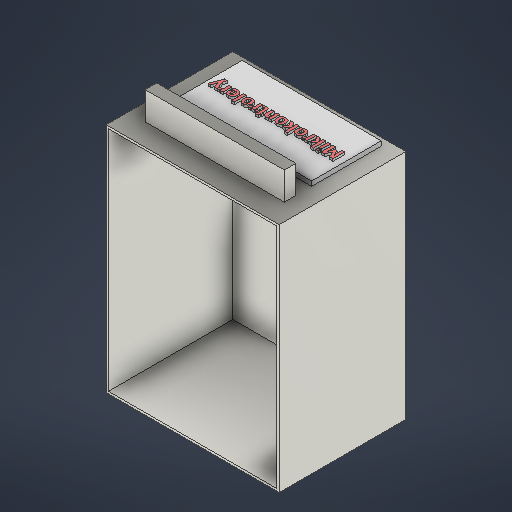
# Autodesk Inventor part: shelf
Saved by Autodesk Inventor 2027 (Build 310192060, 192F)
## iProperties
Created: 2026-06-08
Part Number: shelf
Material: Ogólny
Document SubType Name: Modeling
Designer: User
Density: 1 g/cm^3
Appearance: Domyślna
Author: User
Autodesk Inventor part; units mm, degrees
ref_plane "YZ Plane" through (0, 0, 0) normal (1, 0, 0) x (0, 1, 0)
ref_plane "XZ Plane" through (0, 0, 0) normal (0, 1, 0) x (-1, 0, 0)
ref_plane "XY Plane" through (0, 0, 0) normal (0, 0, 1) x (1, 0, 0)
sketch "Szkic1" plane through (0, 0, 0) normal (0, 1, 0) x (-1, 0, 0)
  line L0 (-37.3, -27.3) -> (37.3, -27.3)
  line L1 (37.3, -27.3) -> (37.3, 27.3)
  line L2 (37.3, 27.3) -> (-37.3, 27.3)
  line L3 (-37.3, 27.3) -> (-37.3, -27.3)
  line L4 (-37.3, -27.3) -> (37.3, 27.3) construction
  line L5 (37.3, -27.3) -> (-37.3, 27.3) construction
  point P0 (0, 0)
  dimension "d0" = 74.6
  dimension "d1" = 54.6
  constraints: 12 end point, 2 midpoint, 2 parallel, 1 horizontal, 1 perpendicular
  measures "d0" distance of L2.end L1.end
  measures "d1" distance of L1.end L0.end
extrude "Wyciągnięcie proste1" add sketch "Szkic1" along normal blind 100
shell "Skorupa1" thickness 1 removed faces 1 at (-12.4333, 33.3333, 27.3)
sketch "Szkic2" plane through (0, 100, 0) normal (0, 1, 0) x (1, 0, 0)
  line L0 (-37.3, -27.3) -> (37.3, -27.3) projected
  line L1 (0, -27.3) -> (0, -15.3)
  line L2 (30, -17.8) -> (-30, -17.8)
  line L3 (-30, -17.8) -> (-30, -12.8)
  line L4 (-30, -12.8) -> (30, -12.8)
  line L5 (30, -12.8) -> (30, -17.8)
  line L6 (30, -17.8) -> (-30, -12.8) construction
  line L7 (-30, -17.8) -> (30, -12.8) construction
  point P0 (0, 0)
  dimension "d5" = 12
  dimension "d6" = 60
  dimension "d7" = 5
  constraints: 14 end point, 3 midpoint, 2 parallel, 1 horizontal, 1 perpendicular, 1 vertical
  measures "d5" distance of L1.start L1.end
  measures "d6" distance of L2.start L2.end
  measures "d7" distance of L2.end L3.end
extrude "Wyciągnięcie proste2" add sketch "Szkic2" along normal blind 12
sketch "Szkic3" plane through (0, 100, 0) normal (0, 1, 0) x (1, 0, 0)
  line L0 (0, 0) -> (0, 9)
  line L1 (30, 24) -> (-30, 24)
  line L2 (-30, 24) -> (-30, -6)
  line L3 (-30, -6) -> (30, -6)
  line L4 (30, -6) -> (30, 24)
  line L5 (30, 24) -> (-30, -6) construction
  line L6 (-30, 24) -> (30, -6) construction
  dimension "d10" = 9
  dimension "d11" = 60
  dimension "d12" = 30
  constraints: 14 end point, 2 midpoint, 2 parallel, 1 horizontal, 1 perpendicular, 1 vertical
  measures "d10" distance of L0.start L0.end
  measures "d11" distance of L3.end L2.end
  measures "d12" distance of L2.end L1.end
extrude "Wyciągnięcie proste3" add sketch "Szkic3" along normal blind 2
sketch "Szkic4" plane through (0, 102, 0) normal (0, 1, 0) x (1, 0, 0)
  line L0 (30, -6) -> (-30, -6) construction
  line L1 (-30, -6) -> (-30, 24) construction
  line L2 (-30, 24) -> (30, 24) construction
  line L3 (30, 24) -> (30, -6) construction
  line L4 (-30, -6) -> (30, -6) projected
  line L5 (-30, 24) -> (-30, -6) projected
  line L6 (30, -6) -> (-30, -6)
  line L7 (-30, -6) -> (-30, 24)
  line L8 (-30, 24) -> (30, 24)
  line L9 (30, 24) -> (30, -6)
  line L10 (22.1617, 10.9226) -> (23.4096, 10.9226)
  line L11 (23.4096, 10.9226) -> (23.4096, 7.6082)
  line L12 (23.4096, 7.6082) -> (24.3173, 9.7476)
  line L13 (24.3173, 9.7476) -> (25.1763, 9.7476)
  line L14 (25.1763, 9.7476) -> (26.0839, 7.6082)
  line L15 (26.0839, 7.6082) -> (26.0839, 10.9226)
  line L16 (26.0839, 10.9226) -> (27.267, 10.9226)
  line L17 (27.267, 10.9226) -> (27.267, 5.9226)
  line L18 (27.267, 5.9226) -> (25.8205, 5.9226)
  line L19 (25.8205, 5.9226) -> (24.7103, 8.3902)
  line L20 (24.7103, 8.3902) -> (23.6082, 5.9226)
  line L21 (23.6082, 5.9226) -> (22.1617, 5.9226)
  line L22 (22.1617, 5.9226) -> (22.1617, 10.9226)
  line L23 (20.0182, 10.9226) -> (21.1933, 10.9226)
  line L24 (21.1933, 10.9226) -> (21.1933, 7.1503)
  line L25 (21.1933, 7.1503) -> (20.0182, 7.1503)
  line L26 (20.0182, 7.1503) -> (20.0182, 10.9226)
  line L27 (19.9818, 6.6114) -> (21.2257, 6.6114)
  line L28 (21.2257, 6.6114) -> (21.2257, 5.6957)
  line L29 (21.2257, 5.6957) -> (19.9818, 5.6957)
  line L30 (19.9818, 5.6957) -> (19.9818, 6.6114)
  line L31 (15.3424, 10.9226) -> (16.7403, 10.9226)
  line L32 (16.7403, 10.9226) -> (17.7613, 9.2857)
  line L33 (17.7613, 9.2857) -> (17.9437, 9.5288)
  line L34 (17.9437, 9.5288) -> (17.9437, 10.9226)
  line L35 (17.9437, 10.9226) -> (19.1187, 10.9226)
  line L36 (19.1187, 10.9226) -> (19.1187, 5.6998)
  line L37 (19.1187, 5.6998) -> (17.9437, 5.6998)
  line L38 (17.9437, 5.6998) -> (17.9437, 8.6252)
  line L39 (17.9437, 8.6252) -> (16.8294, 7.1503)
  line L40 (16.8294, 7.1503) -> (15.4396, 7.1503)
  line L41 (15.4396, 7.1503) -> (16.7605, 8.7751)
  line L42 (16.7605, 8.7751) -> (15.3424, 10.9226)
  line L43 (12.4412, 8.2646) -> (12.5385, 8.2646)
  spline S0 degree 2 poles (12.5385, 8.2646) (12.6074, 8.2403) (12.8626, 8.216) (13.0166, 8.216) knots 0 0 0 1 2 2 2
  spline S1 degree 2 poles (13.0166, 8.216) (13.1989, 8.216) (13.6082, 8.3254) (13.7986, 8.3983) knots 0 0 0 1 2 2 2
  line L44 (13.7986, 8.3983) -> (13.7986, 10.9226)
  line L45 (13.7986, 10.9226) -> (14.9737, 10.9226)
  line L46 (14.9737, 10.9226) -> (14.9737, 7.1503)
  line L47 (14.9737, 7.1503) -> (13.7986, 7.1503)
  line L48 (13.7986, 7.1503) -> (13.7986, 7.6933)
  spline S2 degree 2 poles (13.7986, 7.6933) (13.7176, 7.6203) (13.434, 7.3934) (13.3165, 7.3246) knots 0 0 0 1 2 2 2
  spline S3 degree 2 poles (13.3165, 7.3246) (13.1868, 7.2476) (12.8464, 7.1382) (12.6965, 7.1382) knots 0 0 0 1 2 2 2
  spline S4 degree 2 poles (12.6965, 7.1382) (12.6398, 7.1382) (12.498, 7.1463) (12.4412, 7.1503) knots 0 0 0 1 2 2 2
  line L49 (12.4412, 7.1503) -> (12.4412, 8.2646)
  spline S5 degree 2 poles (8.3732, 9.0385) (8.3732, 9.9704) (9.3902, 11.0401) (10.3181, 11.0401) knots 0 0 0 1 2 2 2
  spline S6 degree 2 poles (10.3181, 11.0401) (11.2419, 11.0401) (12.267, 9.9704) (12.267, 9.0385) knots 0 0 0 1 2 2 2
  spline S7 degree 2 poles (12.267, 9.0385) (12.267, 8.0985) (11.2419, 7.0328) (10.3181, 7.0328) knots 0 0 0 1 2 2 2
  spline S8 degree 2 poles (10.3181, 7.0328) (9.3942, 7.0328) (8.3732, 8.1025) (8.3732, 9.0385) knots 0 0 0 1 2 2 2
  spline S9 degree 2 poles (9.5766, 9.0466) (9.5766, 8.7103) (9.686, 8.2605) (9.7832, 8.1268) knots 0 0 0 1 2 2 2
  spline S10 degree 2 poles (9.7832, 8.1268) (9.8886, 7.985) (10.1519, 7.8756) (10.3181, 7.8756) knots 0 0 0 1 2 2 2
  spline S11 degree 2 poles (10.3181, 7.8756) (10.4801, 7.8756) (10.7354, 7.9729) (10.8408, 8.1106) knots 0 0 0 1 2 2 2
  spline S12 degree 2 poles (10.8408, 8.1106) (10.9421, 8.2403) (11.0636, 8.6981) (11.0636, 9.0466) knots 0 0 0 1 2 2 2
  spline S13 degree 2 poles (11.0636, 9.0466) (11.0636, 9.391) (10.9502, 9.8165) (10.857, 9.9461) knots 0 0 0 1 2 2 2
  spline S14 degree 2 poles (10.857, 9.9461) (10.7638, 10.0758) (10.4801, 10.1973) (10.31, 10.1973) knots 0 0 0 1 2 2 2
  spline S15 degree 2 poles (10.31, 10.1973) (10.1682, 10.1973) (9.8764, 10.0758) (9.7873, 9.9542) knots 0 0 0 1 2 2 2
  spline S16 degree 2 poles (9.7873, 9.9542) (9.686, 9.8124) (9.5766, 9.4032) (9.5766, 9.0466) knots 0 0 0 1 2 2 2
  line L50 (3.9729, 10.9226) -> (5.3707, 10.9226)
  line L51 (5.3707, 10.9226) -> (6.3918, 9.2857)
  line L52 (6.3918, 9.2857) -> (6.5741, 9.5288)
  line L53 (6.5741, 9.5288) -> (6.5741, 10.9226)
  line L54 (6.5741, 10.9226) -> (7.7492, 10.9226)
  line L55 (7.7492, 10.9226) -> (7.7492, 5.6998)
  line L56 (7.7492, 5.6998) -> (6.5741, 5.6998)
  line L57 (6.5741, 5.6998) -> (6.5741, 8.6252)
  line L58 (6.5741, 8.6252) -> (5.4599, 7.1503)
  line L59 (5.4599, 7.1503) -> (4.0701, 7.1503)
  line L60 (4.0701, 7.1503) -> (5.391, 8.7751)
  line L61 (5.391, 8.7751) -> (3.9729, 10.9226)
  spline S17 degree 2 poles (-0.0142, 9.0385) (-0.0142, 9.9704) (1.0028, 11.0401) (1.9307, 11.0401) knots 0 0 0 1 2 2 2
  spline S18 degree 2 poles (1.9307, 11.0401) (2.8545, 11.0401) (3.8797, 9.9704) (3.8797, 9.0385) knots 0 0 0 1 2 2 2
  spline S19 degree 2 poles (3.8797, 9.0385) (3.8797, 8.0985) (2.8545, 7.0328) (1.9307, 7.0328) knots 0 0 0 1 2 2 2
  spline S20 degree 2 poles (1.9307, 7.0328) (1.0069, 7.0328) (-0.0142, 8.1025) (-0.0142, 9.0385) knots 0 0 0 1 2 2 2
  spline S21 degree 2 poles (1.1892, 9.0466) (1.1892, 8.7103) (1.2986, 8.2605) (1.3959, 8.1268) knots 0 0 0 1 2 2 2
  spline S22 degree 2 poles (1.3959, 8.1268) (1.5012, 7.985) (1.7646, 7.8756) (1.9307, 7.8756) knots 0 0 0 1 2 2 2
  spline S23 degree 2 poles (1.9307, 7.8756) (2.0928, 7.8756) (2.3481, 7.9729) (2.4534, 8.1106) knots 0 0 0 1 2 2 2
  spline S24 degree 2 poles (2.4534, 8.1106) (2.5547, 8.2403) (2.6763, 8.6981) (2.6763, 9.0466) knots 0 0 0 1 2 2 2
  spline S25 degree 2 poles (2.6763, 9.0466) (2.6763, 9.391) (2.5628, 9.8165) (2.4696, 9.9461) knots 0 0 0 1 2 2 2
  spline S26 degree 2 poles (2.4696, 9.9461) (2.3764, 10.0758) (2.0928, 10.1973) (1.9226, 10.1973) knots 0 0 0 1 2 2 2
  spline S27 degree 2 poles (1.9226, 10.1973) (1.7808, 10.1973) (1.4891, 10.0758) (1.3999, 9.9542) knots 0 0 0 1 2 2 2
  spline S28 degree 2 poles (1.3999, 9.9542) (1.2986, 9.8124) (1.1892, 9.4032) (1.1892, 9.0466) knots 0 0 0 1 2 2 2
  line L62 (-4.1673, 10.9226) -> (-2.9842, 10.9226)
  line L63 (-2.9842, 10.9226) -> (-2.9842, 9.0547)
  spline S29 degree 2 poles (-2.9842, 9.0547) (-2.9842, 8.8237) (-2.9477, 8.3699) (-2.8991, 8.2646) knots 0 0 0 1 2 2 2
  spline S30 degree 2 poles (-2.8991, 8.2646) (-2.8383, 8.1349) (-2.6114, 8.0255) (-2.4169, 8.0255) knots 0 0 0 1 2 2 2
  spline S31 degree 2 poles (-2.4169, 8.0255) (-2.2751, 8.0255) (-1.9793, 8.1349) (-1.8132, 8.2524) knots 0 0 0 1 2 2 2
  line L64 (-1.8132, 8.2524) -> (-1.8132, 10.9226)
  line L65 (-1.8132, 10.9226) -> (-0.6382, 10.9226)
  line L66 (-0.6382, 10.9226) -> (-0.6382, 7.1503)
  line L67 (-0.6382, 7.1503) -> (-1.8132, 7.1503)
  line L68 (-1.8132, 7.1503) -> (-1.8132, 7.5677)
  spline S32 degree 2 poles (-1.8132, 7.5677) (-2.1009, 7.3246) (-2.6479, 7.049) (-2.9801, 7.049) knots 0 0 0 1 2 2 2
  spline S33 degree 2 poles (-2.9801, 7.049) (-3.5555, 7.049) (-4.1673, 7.7784) (-4.1673, 8.4672) knots 0 0 0 1 2 2 2
  line L69 (-4.1673, 8.4672) -> (-4.1673, 10.9226)
  spline S34 degree 2 poles (-6.481, 10.9955) (-5.7638, 10.9955) (-5.1074, 10.404) (-5.1074, 9.7314) knots 0 0 0 1 2 2 2
  line L70 (-5.1074, 9.7314) -> (-5.1074, 7.9688)
  line L71 (-5.1074, 7.9688) -> (-4.6576, 7.9688)
  line L72 (-4.6576, 7.9688) -> (-4.6576, 7.1503)
  line L73 (-4.6576, 7.1503) -> (-5.1074, 7.1503)
  line L74 (-5.1074, 7.1503) -> (-5.1074, 6.0725)
  line L75 (-5.1074, 6.0725) -> (-6.2824, 6.0725)
  line L76 (-6.2824, 6.0725) -> (-6.2824, 7.1503)
  line L77 (-6.2824, 7.1503) -> (-7.4169, 7.1503)
  line L78 (-7.4169, 7.1503) -> (-7.4169, 7.9688)
  line L79 (-7.4169, 7.9688) -> (-6.2824, 7.9688)
  line L80 (-6.2824, 7.9688) -> (-6.2824, 9.31)
  spline S35 degree 2 poles (-6.2824, 9.31) (-6.2824, 9.5085) (-6.2905, 9.8043) (-6.3391, 9.9218) knots 0 0 0 1 2 2 2
  spline S36 degree 2 poles (-6.3391, 9.9218) (-6.3878, 10.0393) (-6.6268, 10.1771) (-6.8537, 10.1771) knots 0 0 0 1 2 2 2
  spline S37 degree 2 poles (-6.8537, 10.1771) (-6.951, 10.1771) (-7.2549, 10.096) (-7.3156, 10.0636) knots 0 0 0 1 2 2 2
  line L81 (-7.3156, 10.0636) -> (-7.4169, 10.0636)
  line L82 (-7.4169, 10.0636) -> (-7.4169, 10.8902)
  spline S38 degree 2 poles (-7.4169, 10.8902) (-7.2265, 10.9388) (-6.797, 10.9955) (-6.481, 10.9955) knots 0 0 0 1 2 2 2
  line L83 (-10.4275, 8.2646) -> (-10.3302, 8.2646)
  spline S39 degree 2 poles (-10.3302, 8.2646) (-10.2613, 8.2403) (-10.0061, 8.216) (-9.8521, 8.216) knots 0 0 0 1 2 2 2
  spline S40 degree 2 poles (-9.8521, 8.216) (-9.6698, 8.216) (-9.2605, 8.3254) (-9.0701, 8.3983) knots 0 0 0 1 2 2 2
  line L84 (-9.0701, 8.3983) -> (-9.0701, 10.9226)
  line L85 (-9.0701, 10.9226) -> (-7.8951, 10.9226)
  line L86 (-7.8951, 10.9226) -> (-7.8951, 7.1503)
  line L87 (-7.8951, 7.1503) -> (-9.0701, 7.1503)
  line L88 (-9.0701, 7.1503) -> (-9.0701, 7.6933)
  spline S41 degree 2 poles (-9.0701, 7.6933) (-9.1511, 7.6203) (-9.4348, 7.3934) (-9.5523, 7.3246) knots 0 0 0 1 2 2 2
  spline S42 degree 2 poles (-9.5523, 7.3246) (-9.6819, 7.2476) (-10.0223, 7.1382) (-10.1722, 7.1382) knots 0 0 0 1 2 2 2
  spline S43 degree 2 poles (-10.1722, 7.1382) (-10.2289, 7.1382) (-10.3707, 7.1463) (-10.4275, 7.1503) knots 0 0 0 1 2 2 2
  line L89 (-10.4275, 7.1503) -> (-10.4275, 8.2646)
  spline S44 degree 2 poles (-14.4955, 9.0385) (-14.4955, 9.9704) (-13.4785, 11.0401) (-12.5506, 11.0401) knots 0 0 0 1 2 2 2
  spline S45 degree 2 poles (-12.5506, 11.0401) (-11.6268, 11.0401) (-10.6017, 9.9704) (-10.6017, 9.0385) knots 0 0 0 1 2 2 2
  spline S46 degree 2 poles (-10.6017, 9.0385) (-10.6017, 8.0985) (-11.6268, 7.0328) (-12.5506, 7.0328) knots 0 0 0 1 2 2 2
  spline S47 degree 2 poles (-12.5506, 7.0328) (-13.4745, 7.0328) (-14.4955, 8.1025) (-14.4955, 9.0385) knots 0 0 0 1 2 2 2
  spline S48 degree 2 poles (-13.2921, 9.0466) (-13.2921, 8.7103) (-13.1827, 8.2605) (-13.0855, 8.1268) knots 0 0 0 1 2 2 2
  spline S49 degree 2 poles (-13.0855, 8.1268) (-12.9801, 7.985) (-12.7168, 7.8756) (-12.5506, 7.8756) knots 0 0 0 1 2 2 2
  spline S50 degree 2 poles (-12.5506, 7.8756) (-12.3886, 7.8756) (-12.1333, 7.9729) (-12.028, 8.1106) knots 0 0 0 1 2 2 2
  spline S51 degree 2 poles (-12.028, 8.1106) (-11.9267, 8.2403) (-11.8051, 8.6981) (-11.8051, 9.0466) knots 0 0 0 1 2 2 2
  spline S52 degree 2 poles (-11.8051, 9.0466) (-11.8051, 9.391) (-11.9186, 9.8165) (-12.0118, 9.9461) knots 0 0 0 1 2 2 2
  spline S53 degree 2 poles (-12.0118, 9.9461) (-12.1049, 10.0758) (-12.3886, 10.1973) (-12.5588, 10.1973) knots 0 0 0 1 2 2 2
  spline S54 degree 2 poles (-12.5588, 10.1973) (-12.7006, 10.1973) (-12.9923, 10.0758) (-13.0814, 9.9542) knots 0 0 0 1 2 2 2
  spline S55 degree 2 poles (-13.0814, 9.9542) (-13.1827, 9.8124) (-13.2921, 9.4032) (-13.2921, 9.0466) knots 0 0 0 1 2 2 2
  line L90 (-16.2946, 10.9226) -> (-15.1195, 10.9226)
  line L91 (-15.1195, 10.9226) -> (-15.1195, 5.6998)
  line L92 (-15.1195, 5.6998) -> (-16.2946, 5.6998)
  line L93 (-16.2946, 5.6998) -> (-16.2946, 10.9226)
  spline S56 degree 2 poles (-19.1268, 11.0239) (-18.0571, 11.0239) (-16.9186, 10.0028) (-16.9186, 9.0588) knots 0 0 0 1 2 2 2
  spline S57 degree 2 poles (-16.9186, 9.0588) (-16.9186, 8.1349) (-17.9801, 7.0328) (-18.9364, 7.0328) knots 0 0 0 1 2 2 2
  spline S58 degree 2 poles (-18.9364, 7.0328) (-19.7994, 7.0328) (-20.6746, 7.9688) (-20.6746, 8.8359) knots 0 0 0 1 2 2 2
  line L94 (-20.6746, 8.8359) -> (-20.6746, 9.2613)
  line L95 (-20.6746, 9.2613) -> (-18.0936, 9.2613)
  spline S59 degree 2 poles (-18.0936, 9.2613) (-18.1098, 9.5247) (-18.3002, 9.8732) (-18.4542, 9.9785) knots 0 0 0 1 2 2 2
  spline S60 degree 2 poles (-18.4542, 9.9785) (-18.6041, 10.0839) (-19.0093, 10.173) (-19.2484, 10.173) knots 0 0 0 1 2 2 2
  spline S61 degree 2 poles (-19.2484, 10.173) (-19.451, 10.173) (-19.8481, 10.0839) (-20.0142, 10.0069) knots 0 0 0 1 2 2 2
  spline S62 degree 2 poles (-20.0142, 10.0069) (-20.16, 9.9461) (-20.4032, 9.7962) (-20.4801, 9.7395) knots 0 0 0 1 2 2 2
  line L96 (-20.4801, 9.7395) -> (-20.6058, 9.7395)
  line L97 (-20.6058, 9.7395) -> (-20.6058, 10.7119)
  spline S63 degree 2 poles (-20.6058, 10.7119) (-20.4599, 10.7686) (-20.2249, 10.8659) (-20.0142, 10.9145) knots 0 0 0 1 2 2 2
  spline S64 degree 2 poles (-20.0142, 10.9145) (-19.8237, 10.9672) (-19.4186, 11.0239) (-19.1268, 11.0239) knots 0 0 0 1 2 2 2
  spline S65 degree 2 poles (-19.5158, 8.5523) (-19.5077, 8.1795) (-19.1795, 7.7865) (-18.8432, 7.7865) knots 0 0 0 1 2 2 2
  spline S66 degree 2 poles (-18.8432, 7.7865) (-18.4988, 7.7865) (-18.1098, 8.1998) (-18.0895, 8.5523) knots 0 0 0 1 2 2 2
  line L98 (-18.0895, 8.5523) -> (-19.5158, 8.5523)
  line L99 (-23.8108, 8.2646) -> (-23.7135, 8.2646)
  spline S67 degree 2 poles (-23.7135, 8.2646) (-23.6447, 8.2403) (-23.3894, 8.216) (-23.2354, 8.216) knots 0 0 0 1 2 2 2
  spline S68 degree 2 poles (-23.2354, 8.216) (-23.0531, 8.216) (-22.6438, 8.3254) (-22.4534, 8.3983) knots 0 0 0 1 2 2 2
  line L100 (-22.4534, 8.3983) -> (-22.4534, 10.9226)
  line L101 (-22.4534, 10.9226) -> (-21.2784, 10.9226)
  line L102 (-21.2784, 10.9226) -> (-21.2784, 7.1503)
  line L103 (-21.2784, 7.1503) -> (-22.4534, 7.1503)
  line L104 (-22.4534, 7.1503) -> (-22.4534, 7.6933)
  spline S69 degree 2 poles (-22.4534, 7.6933) (-22.5344, 7.6203) (-22.8181, 7.3934) (-22.9356, 7.3246) knots 0 0 0 1 2 2 2
  spline S70 degree 2 poles (-22.9356, 7.3246) (-23.0652, 7.2476) (-23.4056, 7.1382) (-23.5555, 7.1382) knots 0 0 0 1 2 2 2
  spline S71 degree 2 poles (-23.5555, 7.1382) (-23.6122, 7.1382) (-23.7541, 7.1463) (-23.8108, 7.1503) knots 0 0 0 1 2 2 2
  line L105 (-23.8108, 7.1503) -> (-23.8108, 8.2646)
  line L106 (-27.7776, 7.1503) -> (-25.8772, 12.3043)
  line L107 (-25.8772, 12.3043) -> (-24.613, 12.3043)
  line L108 (-24.613, 12.3043) -> (-25.1844, 10.8294)
  line L109 (-25.1844, 10.8294) -> (-23.8027, 7.1503)
  line L110 (-23.8027, 7.1503) -> (-25.0344, 7.1503)
  line L111 (-25.0344, 7.1503) -> (-25.8286, 9.5166)
  line L112 (-25.8286, 9.5166) -> (-26.5701, 7.1503)
  line L113 (-26.5701, 7.1503) -> (-27.7776, 7.1503)
  point P0 (0, 0)
  dimension "d1" = 54.6
  constraints: 8 end point, 2 coincident, 2 parallel, 1 horizontal, 1 perpendicular, 2 other
extrude "Wyciągnięcie proste4" add sketch "Szkic4" along normal blind 1 contours L10 L11 L12 L13 L14 L15 L16 L17 L18 L19 L20 L21 L22 | L23 L24 L25 L26 | L27 L28 L29 L30 | L31 L32 L33 L34 L35 L36 L37 L38 L39 L40 L41 L42 | L43 S0 S1 L44 L45 L46 L47 L48 S2 S3 S4 L49 | S5 S6 S7 S8 | L50 L51 L52 L53 L54 L55 L56 L57 L58 L59 L60 L61 | S17 S18 S19 S20 | L62 L63 S29 S30 S31 L64 L65 L66 L67 L68 S32 S33 L69 | S34 L70 L71 L72 L73 L74 L75 L76 L77 L78 L79 L80 S35 S36 S37 L81 L82 S38 | L83 S39 S40 L84 L85 L86 L87 L88 S41 S42 S43 L89 | S44 S45 S46 S47 | L90 L91 L92 L93 | S56 S57 S58 L94 L95 S59 S60 S61 S62 L96 L97 S63 S64 | L99 S67 S68 L100 L101 L102 L103 L104 S69 S70 S71 L109 L105 | L109 S71 L105 | L105 L110 L111 L112 L113 L106 L107 L108 L109
